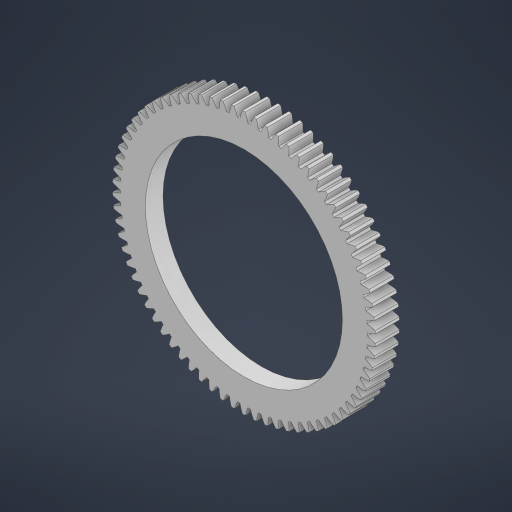
# Autodesk Inventor part: Ring Gear Base
Saved by Autodesk Inventor 2023 (Build 270158000, 158)
## iProperties
Created: 2023-08-11
Part Number: Ring Gear Base
Material: Generic
Document SubType Name: Modeling
Designer: Izack Waczko
Density: 1 g/cm^3
Appearance: Default
Author: Izack Waczko
Autodesk Inventor part; units mm, degrees
ref_plane "YZ Plane" through (0, 0, 0) normal (1, 0, 0) x (0, 1, 0)
ref_plane "XZ Plane" through (0, 0, 0) normal (0, 1, 0) x (-1, 0, 0)
ref_plane "XY Plane" through (0, 0, 0) normal (0, 0, 1) x (1, 0, 0)
sketch "Sketch1" plane through (0, 0, 0) normal (0, 0, 1) x (1, 0, 0)
  line L0 (-44.3976, 4.5) -> (-44.3976, -4.5) construction
  line L1 (3.4024, -4.5) -> (3.4024, 4.5) construction
  line L2 (3.4024, 0) -> (-44.3976, 0) construction
  circle A0 centre (-20.4976, 0) radius 28.5
  circle A1 centre (-20.4976, 0) radius 38.5
  point P0 (0, 0)
  dimension "d0" = 57
  dimension "d1" = 10
  constraints: 3 midpoint, 2 centre point, 2 end point
  measures "d0" diameter of A0
  measures "d1" radial gap between concentric circles of A0 A1
extrude "Extrusion1" add sketch "Sketch1" along normal blind 7
sketch "Sketch2" plane through (-20.4976, 0, 0) normal (0, 0, -1) x (-1, 0, 0)
  circle A0 centre (0, 0) radius 35.5
  circle A1 centre (0, 0) radius 28.5 projected
  point P0 (-20.4976, 0)
  dimension "d4" = 71
  constraints: 1 centre point
  measures "d4" diameter of A0
extrude "Extrusion2" cut sketch "Sketch2" against normal blind 1.9 contours A0 | A1
spur gear teeth "Spur Gear1" teeth 74 pitch diameter 74 tip diameter 76 root diameter 71.5 face width 8 trims to tip circle yes start plane through (-20.4976, 0, 7) normal (0, 0, 1) x (1, 0, 0)
body "Solid1"
